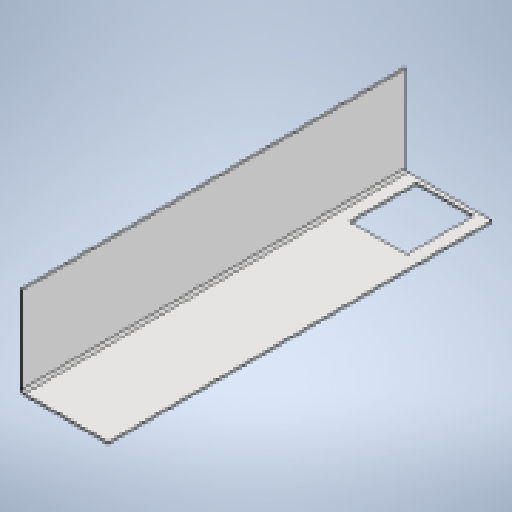
# Autodesk Inventor part: PNS 752 FDS 1200 FLANGE 2
Saved by Autodesk Inventor 2025.1 (Build 291241020, 241B)
## iProperties
Created: 2025-06-24
Part Number: PNS 752 FDS 1200 FLANGE 2
Material: Stainless Steel
Description: DIE16(5)|\ 90°|corrY -___°|X_____|bom___
Document SubType Name: Sheet Metal
Designer: user
Mass: 1762.25 g
Surface Area: 2283.33 cm^2
Volume: 220.281 cm^3
Density: 8 g/cm^3
Sheet Metal Rule: AISI304 2mm Die16
Sheet Metal Width: 0.000 mm
Sheet Metal Length: 0.000 mm
Sheet Metal Area: 0.000 mm^2
Appearance: Default
Author: user
Autodesk Inventor part; units mm, degrees
ref_plane "YZ Plane" through (0, 0, 0) normal (1, 0, 0) x (0, 1, 0)
ref_plane "XZ Plane" through (0, 0, 0) normal (0, 1, 0) x (-1, 0, 0)
ref_plane "XY Plane" through (0, 0, 0) normal (0, 0, 1) x (1, 0, 0)
sketch "Sketch1" plane through (0, 0, 0) normal (0, 0, 1) x (1, 0, 0)
  line L0 (-46, -200) -> (46, -200)
  line L1 (46, -200) -> (46, 200)
  line L2 (46, 200) -> (-46, 200)
  line L3 (-46, 200) -> (-46, -200)
  line L4 (-46, -200) -> (46, 200) construction
  line L5 (46, -200) -> (-46, 200) construction
  point P0 (0, 0)
  dimension "d154" = 92
  dimension "d155" = 400
  measures "d154" distance of L1.end L2.end
  measures "d155" distance of L0.end L1.end
extrude "Plate5" add sketch "Sketch1" along normal blind 2
sketch "Sketch7" plane through (-44, -200, 0) normal (-1, 0, 0) x (0, -1, 0)
  line L0 (-400, 0) -> (0, 0)
  line L1 (0, 0) -> (0, 94)
  line L2 (0, 94) -> (-400, 94)
  line L3 (-400, 94) -> (-400, 0)
  constraints: 6 end point, 1 horizontal, 1 perpendicular, 1 vertical
edge flange "Flange3" height 94 angle 90 thickness 2 bend radius 2.75 thickness toward (-1, 0, 0) relief round relief width 2 relief depth 1 edges at (-46, 0, 2) wall of the first edge with corners at (-44, 200, 0) (-44, -200, 0) (-44, -200, 94) (-44, 200, 94)
bend "Bend3"
corner "Corner3"
sketch "Sketch8" plane through (0, 0, 2) normal (0, 0, 1) x (1, 0, 0)
  line L0 (46, 200) -> (46, -200) projected
  line L1 (-41.25, 200) -> (46, 200) projected
  line L2 (32.375, 195) -> (-27.625, 195)
  line L3 (-27.625, 195) -> (-27.625, 125)
  line L4 (-27.625, 125) -> (32.375, 125)
  line L5 (32.375, 125) -> (32.375, 195)
  line L6 (32.375, 195) -> (-27.625, 125) construction
  line L7 (-27.625, 195) -> (32.375, 125) construction
  point P0 (0, 0)
  point P1 (2.375, 160)
  point P2 (2.375, 200)
  dimension "d167" = 60
  dimension "d168" = 70
  dimension "d169" = 5
  constraints: 12 end point, 3 midpoint, 2 parallel, 1 horizontal, 1 perpendicular, 1 vertical alignment
  measures "d167" distance of L4.end L3.end
  measures "d168" distance of L3.end L2.end
  measures "d169" distance between parallel lines of L1 L2
extrude "Cut1" cut sketch "Sketch8" against normal blind 2
body "Solid3"
